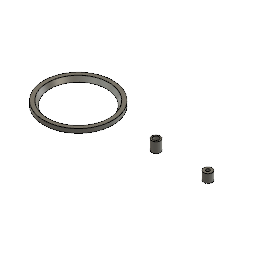
test v5 (Autodesk Fusion 360 design; units mm, degrees)
Autodesk Fusion 360 part; units mm, degrees
sketch "Sketch1" plane through (0, 0, 0) normal (0, 1, 0) x (1, 0, 0)
  circle A0 centre (0, 0) radius 32.5
  circle A1 centre (0, 0) radius 40
  dimension "d1" = 65
  dimension "d2" = 80
  constraint coincident A0.centre A1.centre
  measures "d1" diameter of A0
  measures "d2" diameter of A1
extrude "Extrude1" add sketch "Sketch1" along normal blind 5 makes body 1
chamfer "Chamfer1" distance 3 distance2 5 1 edges at (-30.3006, 5, -11.7525) measured on face at (37.2301, 5, 3.6019) on bodies 1
sketch "Sketch2" plane through (0, 0, 0) normal (0, 1, 0) x (1, 0, 0)
  circle A0 centre (90, 0) radius 5
  dimension "d9" = 10
  measures "d9" diameter of A0
extrude "Extrude2" add sketch "Sketch2" along normal blind 12 separate body makes body 2
sketch "Sketch3" plane through (0, 12, 0) normal (0, 1, 0) x (-1, 0, 0)
  circle A0 centre (-90, 0) radius 5
  circle A1 centre (-90, 0) radius 3.225
  dimension "d12" = 6.45
  constraint concentric A0 A1
  measures "d12" diameter of A1
extrude "Extrude3" cut sketch "Sketch3" against normal blind 10 contours A1 bodies 2
sketch "Sketch4" plane through (0, 0, 0) normal (0, 1, 0) x (1, 0, 0)
  circle A0 centre (150, 0) radius 2
  circle A1 centre (150, 0) radius 5
  dimension "d15" = 4
  dimension "d16" = 10
  constraint concentric A0 A1
  measures "d15" diameter of A0
  measures "d16" diameter of A1
extrude "Extrude4" add sketch "Sketch4" along normal blind 10 separate body makes body 3
